Autodesk Inventor part; units mm, degrees
(part 4 of 4)
sketch "Sketch3" plane through (-107.46, -92.5006, 10.9251) normal (0, 0, 1) x (1, 0, 0)
  circle A0 centre (-216.125, 0) radius 1.35
  circle A1 centre (-216.125, 57) radius 1.35
  circle A2 centre (-216.125, -57) radius 1.35
  circle A3 centre (-216.125, 57) radius 1.35
  circle A4 centre (-216.125, 0) radius 1.35
  circle A5 centre (-216.125, -57) radius 1.35
  circle A6 centre (-175.75, 14.25) radius 1.35
  circle A7 centre (-175.75, -23.75) radius 1.35
  circle A8 centre (-133.753, -57) radius 1.35
  circle A9 centre (-114, 14.25) radius 1.35
  circle A10 centre (-73.625, 57) radius 1.35
  circle A11 centre (-66.5, -19) radius 1.35
  circle A12 centre (-47.5, -57) radius 1.35
  circle A13 centre (-45.125, 11.875) radius 1.35
  line L0 (-205.2313, 59.21) -> (-211.6644, 41.535)
  line L1 (-211.6644, 41.535) -> (-209.1644, 41.535)
  line L2 (-209.1644, 41.535) -> (-202.7313, 59.21)
  line L3 (-202.7313, 59.21) -> (-205.2313, 59.21)
  line L4 (-195.2313, 59.21) -> (-201.6644, 41.535)
  line L5 (-201.6644, 41.535) -> (-199.1644, 41.535)
  line L6 (-199.1644, 41.535) -> (-192.7313, 59.21)
  line L7 (-192.7313, 59.21) -> (-195.2313, 59.21)
  line L8 (-185.2313, 59.21) -> (-191.6644, 41.535)
  line L9 (-191.6644, 41.535) -> (-189.1644, 41.535)
  line L10 (-189.1644, 41.535) -> (-182.7313, 59.21)
  line L11 (-182.7313, 59.21) -> (-185.2313, 59.21)
  line L12 (-175.2313, 59.21) -> (-181.6644, 41.535)
  line L13 (-181.6644, 41.535) -> (-179.1644, 41.535)
  line L14 (-179.1644, 41.535) -> (-172.7313, 59.21)
  line L15 (-172.7313, 59.21) -> (-175.2313, 59.21)
  line L16 (-165.2313, 59.21) -> (-171.6644, 41.535)
  line L17 (-171.6644, 41.535) -> (-169.1644, 41.535)
  line L18 (-169.1644, 41.535) -> (-162.7313, 59.21)
  line L19 (-162.7313, 59.21) -> (-165.2313, 59.21)
  line L20 (-155.2313, 59.21) -> (-161.6644, 41.535)
  line L21 (-161.6644, 41.535) -> (-159.1644, 41.535)
  line L22 (-159.1644, 41.535) -> (-152.7313, 59.21)
  line L23 (-152.7313, 59.21) -> (-155.2313, 59.21)
  line L24 (-145.2313, 59.21) -> (-151.6644, 41.535)
  line L25 (-151.6644, 41.535) -> (-149.1644, 41.535)
  line L26 (-149.1644, 41.535) -> (-142.7313, 59.21)
  line L27 (-142.7313, 59.21) -> (-145.2313, 59.21)
  line L28 (-135.2313, 59.21) -> (-141.6644, 41.535)
  line L29 (-141.6644, 41.535) -> (-139.1644, 41.535)
  line L30 (-139.1644, 41.535) -> (-132.7313, 59.21)
  line L31 (-132.7313, 59.21) -> (-135.2313, 59.21)
  line L32 (-136.6647, 41.535) -> (-134.1647, 41.535)
  line L33 (-134.1647, 41.535) -> (-131.39, 49.1583)
  line L34 (-131.39, 49.1583) -> (-131.39, 56.027)
  line L35 (-131.39, 56.027) -> (-136.6647, 41.535)
  line L36 (-143.77, 35.75) -> (-141.27, 35.75)
  line L37 (-141.27, 35.75) -> (-139.8378, 39.685)
  line L38 (-139.8378, 39.685) -> (-142.3378, 39.685)
  line L39 (-142.3378, 39.685) -> (-143.77, 35.75)
  line L40 (-153.77, 35.75) -> (-151.27, 35.75)
  line L41 (-151.27, 35.75) -> (-149.8378, 39.685)
  line L42 (-149.8378, 39.685) -> (-152.3378, 39.685)
  line L43 (-152.3378, 39.685) -> (-153.77, 35.75)
  line L44 (-163.77, 35.75) -> (-161.27, 35.75)
  line L45 (-161.27, 35.75) -> (-159.8378, 39.685)
  line L46 (-159.8378, 39.685) -> (-162.3378, 39.685)
  line L47 (-162.3378, 39.685) -> (-163.77, 35.75)
  line L48 (-173.77, 35.75) -> (-171.27, 35.75)
  line L49 (-171.27, 35.75) -> (-169.8378, 39.685)
  line L50 (-169.8378, 39.685) -> (-172.3378, 39.685)
  line L51 (-172.3378, 39.685) -> (-173.77, 35.75)
  line L52 (-183.77, 35.75) -> (-181.27, 35.75)
  line L53 (-181.27, 35.75) -> (-179.8378, 39.685)
  line L54 (-179.8378, 39.685) -> (-182.3378, 39.685)
  line L55 (-182.3378, 39.685) -> (-183.77, 35.75)
  line L56 (-193.77, 35.75) -> (-191.27, 35.75)
  line L57 (-191.27, 35.75) -> (-189.8378, 39.685)
  line L58 (-189.8378, 39.685) -> (-192.3378, 39.685)
  line L59 (-192.3378, 39.685) -> (-193.77, 35.75)
  line L60 (-203.77, 35.75) -> (-201.27, 35.75)
  line L61 (-201.27, 35.75) -> (-199.8378, 39.685)
  line L62 (-199.8378, 39.685) -> (-202.3378, 39.685)
  line L63 (-202.3378, 39.685) -> (-203.77, 35.75)
  line L64 (-213.77, 35.75) -> (-211.27, 35.75)
  line L65 (-211.27, 35.75) -> (-209.8378, 39.685)
  line L66 (-209.8378, 39.685) -> (-212.3378, 39.685)
  line L67 (-212.3378, 39.685) -> (-213.77, 35.75)
  line L68 (-208.77, 35.75) -> (-206.27, 35.75)
  line L69 (-206.27, 35.75) -> (-204.8378, 39.685)
  line L70 (-204.8378, 39.685) -> (-207.3378, 39.685)
  line L71 (-207.3378, 39.685) -> (-208.77, 35.75)
  line L72 (-198.77, 35.75) -> (-196.27, 35.75)
  line L73 (-196.27, 35.75) -> (-194.8378, 39.685)
  line L74 (-194.8378, 39.685) -> (-197.3378, 39.685)
  line L75 (-197.3378, 39.685) -> (-198.77, 35.75)
  line L76 (-188.77, 35.75) -> (-186.27, 35.75)
  line L77 (-186.27, 35.75) -> (-184.8378, 39.685)
  line L78 (-184.8378, 39.685) -> (-187.3378, 39.685)
  line L79 (-187.3378, 39.685) -> (-188.77, 35.75)
  line L80 (-178.77, 35.75) -> (-176.27, 35.75)
  line L81 (-176.27, 35.75) -> (-174.8378, 39.685)
  line L82 (-174.8378, 39.685) -> (-177.3378, 39.685)
  line L83 (-177.3378, 39.685) -> (-178.77, 35.75)
  line L84 (-168.77, 35.75) -> (-166.27, 35.75)
  line L85 (-166.27, 35.75) -> (-164.8378, 39.685)
  line L86 (-164.8378, 39.685) -> (-167.3378, 39.685)
  line L87 (-167.3378, 39.685) -> (-168.77, 35.75)
  line L88 (-158.77, 35.75) -> (-156.27, 35.75)
  line L89 (-156.27, 35.75) -> (-154.8378, 39.685)
  line L90 (-154.8378, 39.685) -> (-157.3378, 39.685)
  line L91 (-157.3378, 39.685) -> (-158.77, 35.75)
  line L92 (-148.77, 35.75) -> (-146.27, 35.75)
  line L93 (-146.27, 35.75) -> (-144.8378, 39.685)
  line L94 (-144.8378, 39.685) -> (-147.3378, 39.685)
  line L95 (-147.3378, 39.685) -> (-148.77, 35.75)
  line L96 (-138.7702, 35.75) -> (-136.2702, 35.75)
  line L97 (-136.2702, 35.75) -> (-134.838, 39.685)
  line L98 (-134.838, 39.685) -> (-137.338, 39.685)
  line L99 (-137.338, 39.685) -> (-138.7702, 35.75)
  line L100 (-210.231, 59.21) -> (-213.77, 49.4867)
  line L101 (-213.77, 49.4867) -> (-213.77, 42.618)
  line L102 (-213.77, 42.618) -> (-207.731, 59.21)
  line L103 (-207.731, 59.21) -> (-210.231, 59.21)
  line L104 (-140.2313, 59.21) -> (-146.6644, 41.535)
  line L105 (-146.6644, 41.535) -> (-144.1644, 41.535)
  line L106 (-144.1644, 41.535) -> (-137.7313, 59.21)
  line L107 (-137.7313, 59.21) -> (-140.2313, 59.21)
  line L108 (-150.2313, 59.21) -> (-156.6644, 41.535)
  line L109 (-156.6644, 41.535) -> (-154.1644, 41.535)
  line L110 (-154.1644, 41.535) -> (-147.7313, 59.21)
  line L111 (-147.7313, 59.21) -> (-150.2313, 59.21)
  line L112 (-160.2313, 59.21) -> (-166.6644, 41.535)
  line L113 (-166.6644, 41.535) -> (-164.1644, 41.535)
  line L114 (-164.1644, 41.535) -> (-157.7313, 59.21)
  line L115 (-157.7313, 59.21) -> (-160.2313, 59.21)
  line L116 (-170.2313, 59.21) -> (-176.6644, 41.535)
  line L117 (-176.6644, 41.535) -> (-174.1644, 41.535)
  line L118 (-174.1644, 41.535) -> (-167.7313, 59.21)
  line L119 (-167.7313, 59.21) -> (-170.2313, 59.21)
  line L120 (-180.2313, 59.21) -> (-186.6644, 41.535)
  line L121 (-186.6644, 41.535) -> (-184.1644, 41.535)
  line L122 (-184.1644, 41.535) -> (-177.7313, 59.21)
  line L123 (-177.7313, 59.21) -> (-180.2313, 59.21)
  line L124 (-190.2313, 59.21) -> (-196.6644, 41.535)
  line L125 (-196.6644, 41.535) -> (-194.1644, 41.535)
  line L126 (-194.1644, 41.535) -> (-187.7313, 59.21)
  line L127 (-187.7313, 59.21) -> (-190.2313, 59.21)
  line L128 (-200.2313, 59.21) -> (-206.6644, 41.535)
  line L129 (-206.6644, 41.535) -> (-204.1644, 41.535)
  line L130 (-204.1644, 41.535) -> (-197.7313, 59.21)
  line L131 (-197.7313, 59.21) -> (-200.2313, 59.21)
  line L132 (-133.77, 35.75) -> (-78.7722, 35.75)
  line L133 (-78.7722, 35.75) -> (-77.34, 39.685)
  line L134 (-77.34, 39.685) -> (-132.3378, 39.685)
  line L135 (-132.3378, 39.685) -> (-133.77, 35.75)
  line L136 (-216.125, 61.75) -> (216.125, 61.75)
  arc A14 (220.875, 57) -> (216.125, 61.75) centre (216.125, 57) ccw
  line L137 (220.875, 57) -> (220.875, -57)
  arc A15 (216.125, -61.75) -> (220.875, -57) centre (216.125, -57) ccw
  line L138 (216.125, -61.75) -> (-216.125, -61.75)
  arc A16 (-220.875, -57) -> (-216.125, -61.75) centre (-216.125, -57) ccw
  line L139 (-220.875, -57) -> (-220.875, 57)
  arc A17 (-216.125, 61.75) -> (-220.875, 57) centre (-216.125, 57) ccw
  line L140 (-129.54, 41.535) -> (-77.34, 41.535)
  line L141 (-77.34, 41.535) -> (-77.34, 59.315)
  line L142 (-77.34, 59.315) -> (-129.54, 59.315)
  line L143 (-129.54, 59.315) -> (-129.54, 41.535)
  line L144 (-54.75, 45.25) -> (-54.75, 59.25)
  line L145 (-54.75, 59.25) -> (-68.75, 59.25)
  line L146 (-68.75, 59.25) -> (-68.75, 45.25)
  line L147 (-68.75, 45.25) -> (-54.75, 45.25)
  line L148 (-16.75, 45.25) -> (-16.75, 59.25)
  line L149 (-16.75, 59.25) -> (-30.75, 59.25)
  line L150 (-30.75, 59.25) -> (-30.75, 45.25)
  line L151 (-30.75, 45.25) -> (-16.75, 45.25)
  line L152 (2.25, 45.25) -> (2.25, 59.25)
  line L153 (2.25, 59.25) -> (-11.75, 59.25)
  line L154 (-11.75, 59.25) -> (-11.75, 45.25)
  line L155 (-11.75, 45.25) -> (2.25, 45.25)
  line L156 (21.25, 45.25) -> (21.25, 59.25)
  line L157 (21.25, 59.25) -> (7.25, 59.25)
  line L158 (7.25, 59.25) -> (7.25, 45.25)
  line L159 (7.25, 45.25) -> (21.25, 45.25)
  line L160 (40.25, 45.25) -> (40.25, 59.25)
  line L161 (40.25, 59.25) -> (26.25, 59.25)
  line L162 (26.25, 59.25) -> (26.25, 45.25)
  line L163 (26.25, 45.25) -> (40.25, 45.25)
  line L164 (68.75, 45.25) -> (68.75, 59.25)
  line L165 (68.75, 59.25) -> (54.75, 59.25)
  line L166 (54.75, 59.25) -> (54.75, 45.25)
  line L167 (54.75, 45.25) -> (68.75, 45.25)
  line L168 (87.75, 45.25) -> (87.75, 59.25)
  line L169 (87.75, 59.25) -> (73.75, 59.25)
  line L170 (73.75, 59.25) -> (73.75, 45.25)
  line L171 (73.75, 45.25) -> (87.75, 45.25)
  line L172 (106.75, 45.25) -> (106.75, 59.25)
  line L173 (106.75, 59.25) -> (92.75, 59.25)
  line L174 (92.75, 59.25) -> (92.75, 45.25)
  line L175 (92.75, 45.25) -> (106.75, 45.25)
  line L176 (125.75, 45.25) -> (125.75, 59.25)
  line L177 (125.75, 59.25) -> (111.75, 59.25)
  line L178 (111.75, 59.25) -> (111.75, 45.25)
  line L179 (111.75, 45.25) -> (125.75, 45.25)
  line L180 (154.25, 45.25) -> (154.25, 59.25)
  line L181 (154.25, 59.25) -> (140.25, 59.25)
  line L182 (140.25, 59.25) -> (140.25, 45.25)
  line L183 (140.25, 45.25) -> (154.25, 45.25)
  line L184 (173.25, 45.25) -> (173.25, 59.25)
  line L185 (173.25, 59.25) -> (159.25, 59.25)
  line L186 (159.25, 59.25) -> (159.25, 45.25)
  line L187 (159.25, 45.25) -> (173.25, 45.25)
  line L188 (192.25, 45.25) -> (192.25, 59.25)
  line L189 (192.25, 59.25) -> (178.25, 59.25)
  line L190 (178.25, 59.25) -> (178.25, 45.25)
  line L191 (178.25, 45.25) -> (192.25, 45.25)
  line L192 (211.25, 45.25) -> (211.25, 59.25)
  line L193 (211.25, 59.25) -> (197.25, 59.25)
  line L194 (197.25, 59.25) -> (197.25, 45.25)
  line L195 (197.25, 45.25) -> (211.25, 45.25)
  line L196 (-197.25, 16.75) -> (-197.25, 30.75)
  line L197 (-197.25, 30.75) -> (-211.25, 30.75)
  line L198 (-211.25, 30.75) -> (-211.25, 16.75)
  line L199 (-211.25, 16.75) -> (-197.25, 16.75)
  line L200 (-178.25, 30.75) -> (-192.25, 30.75)
  line L201 (-192.25, 30.75) -> (-192.25, 16.75)
  line L202 (-192.25, 16.75) -> (-178.25, 16.75)
  line L203 (-178.25, 16.75) -> (-178.25, 30.75)
  line L204 (-159.25, 30.75) -> (-173.25, 30.75)
  line L205 (-173.25, 30.75) -> (-173.25, 16.75)
  line L206 (-173.25, 16.75) -> (-159.25, 16.75)
  line L207 (-159.25, 16.75) -> (-159.25, 30.75)
  line L208 (-197.25, 11.75) -> (-211.25, 11.75)
  line L209 (-211.25, 11.75) -> (-211.25, -2.25)
  line L210 (-211.25, -2.25) -> (-197.25, -2.25)
  line L211 (-197.25, -2.25) -> (-197.25, 11.75)
  line L212 (-178.25, 11.75) -> (-192.25, 11.75)
  line L213 (-192.25, 11.75) -> (-192.25, -2.25)
  line L214 (-192.25, -2.25) -> (-178.25, -2.25)
  line L215 (-178.25, -2.25) -> (-178.25, 11.75)
  line L216 (-159.25, 11.75) -> (-173.25, 11.75)
  line L217 (-173.25, 11.75) -> (-173.25, -2.25)
  line L218 (-173.25, -2.25) -> (-159.25, -2.25)
  line L219 (-159.25, -2.25) -> (-159.25, 11.75)
  line L220 (-197.25, -7.25) -> (-211.25, -7.25)
  line L221 (-211.25, -7.25) -> (-211.25, -21.25)
  line L222 (-211.25, -21.25) -> (-197.25, -21.25)
  line L223 (-197.25, -21.25) -> (-197.25, -7.25)
  line L224 (-178.25, -7.25) -> (-192.25, -7.25)
  line L225 (-192.25, -7.25) -> (-192.25, -21.25)
  line L226 (-192.25, -21.25) -> (-178.25, -21.25)
  line L227 (-178.25, -21.25) -> (-178.25, -7.25)
  line L228 (-159.25, -7.25) -> (-173.25, -7.25)
  line L229 (-173.25, -7.25) -> (-173.25, -21.25)
  line L230 (-173.25, -21.25) -> (-159.25, -21.25)
  line L231 (-159.25, -21.25) -> (-159.25, -7.25)
  line L232 (-197.25, -26.25) -> (-211.25, -26.25)
  line L233 (-211.25, -26.25) -> (-211.25, -40.25)
  line L234 (-211.25, -40.25) -> (-197.25, -40.25)
  line L235 (-197.25, -40.25) -> (-197.25, -26.25)
  line L236 (-178.25, -26.25) -> (-192.25, -26.25)
  line L237 (-192.25, -26.25) -> (-192.25, -40.25)
  line L238 (-192.25, -40.25) -> (-178.25, -40.25)
  line L239 (-178.25, -40.25) -> (-178.25, -26.25)
  line L240 (-159.25, -26.25) -> (-173.25, -26.25)
  line L241 (-173.25, -26.25) -> (-173.25, -40.25)
  line L242 (-173.25, -40.25) -> (-159.25, -40.25)
  line L243 (-159.25, -40.25) -> (-159.25, -26.25)
  line L244 (-197.25, -45.25) -> (-211.25, -45.25)
  line L245 (-211.25, -45.25) -> (-211.25, -59.25)
  line L246 (-211.25, -59.25) -> (-197.25, -59.25)
  line L247 (-197.25, -59.25) -> (-197.25, -45.25)
  line L248 (-178.25, -45.25) -> (-192.25, -45.25)
  line L249 (-192.25, -45.25) -> (-192.25, -59.25)
  line L250 (-192.25, -59.25) -> (-178.25, -59.25)
  line L251 (-178.25, -59.25) -> (-178.25, -45.25)
  line L252 (-159.25, -45.25) -> (-173.25, -45.25)
  line L253 (-173.25, -45.25) -> (-173.25, -59.25)
  line L254 (-173.25, -59.25) -> (-159.25, -59.25)
  line L255 (-159.25, -59.25) -> (-159.25, -45.25)
  line L256 (-140.25, 16.75) -> (-140.25, 30.75)
  line L257 (-140.25, 30.75) -> (-154.25, 30.75)
  line L258 (-154.25, 30.75) -> (-154.25, 16.75)
  line L259 (-154.25, 16.75) -> (-140.25, 16.75)
  line L260 (-140.25, -11.75) -> (-140.25, 2.25)
  line L261 (-140.25, 2.25) -> (-154.25, 2.25)
  line L262 (-154.25, 2.25) -> (-154.25, -11.75)
  line L263 (-154.25, -11.75) -> (-140.25, -11.75)
  line L264 (-140.25, -49.75) -> (-140.25, -35.75)
  line L265 (-140.25, -35.75) -> (-154.25, -35.75)
  line L266 (-154.25, -35.75) -> (-154.25, -49.75)
  line L267 (-154.25, -49.75) -> (-140.25, -49.75)
  line L268 (-116.5, -59.25) -> (-116.5, -45.25)
  line L269 (-116.5, -45.25) -> (-130.5, -45.25)
  line L270 (-130.5, -45.25) -> (-130.5, -59.25)
  line L271 (-130.5, -59.25) -> (-116.5, -59.25)
  line L272 (-97.5, -59.25) -> (-97.5, -45.25)
  line L273 (-97.5, -45.25) -> (-111.5, -45.25)
  line L274 (-111.5, -45.25) -> (-111.5, -59.25)
  line L275 (-111.5, -59.25) -> (-97.5, -59.25)
  line L276 (-78.5, -59.25) -> (-78.5, -45.25)
  line L277 (-78.5, -45.25) -> (-92.5, -45.25)
  line L278 (-92.5, -45.25) -> (-92.5, -59.25)
  line L279 (-92.5, -59.25) -> (-78.5, -59.25)
  line L280 (-97.5, -40.25) -> (-97.5, -26.25)
  line L281 (-97.5, -26.25) -> (-111.5, -26.25)
  line L282 (-111.5, -26.25) -> (-111.5, -40.25)
  line L283 (-111.5, -40.25) -> (-97.5, -40.25)
  line L284 (-116.5, 16.75) -> (-116.5, 30.75)
  line L285 (-116.5, 30.75) -> (-130.5, 30.75)
  line L286 (-130.5, 30.75) -> (-130.5, 16.75)
  line L287 (-130.5, 16.75) -> (-116.5, 16.75)
  line L288 (-111.5, 30.75) -> (-111.5, 16.75)
  line L289 (-111.5, 16.75) -> (-97.5, 16.75)
  line L290 (-97.5, 16.75) -> (-97.5, 30.75)
  line L291 (-97.5, 30.75) -> (-111.5, 30.75)
  line L292 (-92.5, 30.75) -> (-92.5, 16.75)
  line L293 (-92.5, 16.75) -> (-78.5, 16.75)
  line L294 (-78.5, 16.75) -> (-78.5, 30.75)
  line L295 (-78.5, 30.75) -> (-92.5, 30.75)
  line L296 (-130.5, 11.75) -> (-130.5, -2.25)
  line L297 (-130.5, -2.25) -> (-116.5, -2.25)
  line L298 (-116.5, -2.25) -> (-116.5, 11.75)
  line L299 (-116.5, 11.75) -> (-130.5, 11.75)
  line L300 (-111.5, 11.75) -> (-111.5, -2.25)
  line L301 (-111.5, -2.25) -> (-97.5, -2.25)
  line L302 (-97.5, -2.25) -> (-97.5, 11.75)
  line L303 (-97.5, 11.75) -> (-111.5, 11.75)
  line L304 (-92.5, 11.75) -> (-92.5, -2.25)
  line L305 (-92.5, -2.25) -> (-78.5, -2.25)
  line L306 (-78.5, -2.25) -> (-78.5, 11.75)
  line L307 (-78.5, 11.75) -> (-92.5, 11.75)
  line L308 (-54.75, 16.75) -> (-54.75, 30.75)
  line L309 (-54.75, 30.75) -> (-68.75, 30.75)
  line L310 (-68.75, 30.75) -> (-68.75, 16.75)
  line L311 (-68.75, 16.75) -> (-54.75, 16.75)
  line L312 (-35.75, 16.75) -> (-35.75, 30.75)
  line L313 (-35.75, 30.75) -> (-49.75, 30.75)
  line L314 (-49.75, 30.75) -> (-49.75, 16.75)
  line L315 (-49.75, 16.75) -> (-35.75, 16.75)
  line L316 (-16.75, 16.75) -> (-16.75, 30.75)
  line L317 (-16.75, 30.75) -> (-30.75, 30.75)
  line L318 (-30.75, 30.75) -> (-30.75, 16.75)
  line L319 (-30.75, 16.75) -> (-16.75, 16.75)
  line L320 (2.25, 16.75) -> (2.25, 30.75)
  line L321 (2.25, 30.75) -> (-11.75, 30.75)
  line L322 (-11.75, 30.75) -> (-11.75, 16.75)
  line L323 (-11.75, 16.75) -> (2.25, 16.75)
  line L324 (21.25, 16.75) -> (21.25, 30.75)
  line L325 (21.25, 30.75) -> (7.25, 30.75)
  line L326 (7.25, 30.75) -> (7.25, 16.75)
  line L327 (7.25, 16.75) -> (21.25, 16.75)
  line L328 (40.25, 16.75) -> (40.25, 30.75)
  line L329 (40.25, 30.75) -> (26.25, 30.75)
  line L330 (26.25, 30.75) -> (26.25, 16.75)
  line L331 (26.25, 16.75) -> (40.25, 16.75)
  line L332 (59.25, 16.75) -> (59.25, 30.75)
  line L333 (59.25, 30.75) -> (45.25, 30.75)
  line L334 (45.25, 30.75) -> (45.25, 16.75)
  line L335 (45.25, 16.75) -> (59.25, 16.75)
  line L336 (78.25, 16.75) -> (78.25, 30.75)
  line L337 (78.25, 30.75) -> (64.25, 30.75)
  line L338 (64.25, 30.75) -> (64.25, 16.75)
  line L339 (64.25, 16.75) -> (78.25, 16.75)
  line L340 (97.25, 16.75) -> (97.25, 30.75)
  line L341 (97.25, 30.75) -> (83.25, 30.75)
  line L342 (83.25, 30.75) -> (83.25, 16.75)
  line L343 (83.25, 16.75) -> (97.25, 16.75)
  line L344 (116.25, 16.75) -> (116.25, 30.75)
  line L345 (116.25, 30.75) -> (102.25, 30.75)
  line L346 (102.25, 30.75) -> (102.25, 16.75)
  line L347 (102.25, 16.75) -> (116.25, 16.75)
  line L348 (135.25, 16.75) -> (135.25, 30.75)
  line L349 (135.25, 30.75) -> (121.25, 30.75)
  line L350 (121.25, 30.75) -> (121.25, 16.75)
  line L351 (121.25, 16.75) -> (135.25, 16.75)
  line L352 (154.25, 16.75) -> (154.25, 30.75)
  line L353 (154.25, 30.75) -> (140.25, 30.75)
  line L354 (140.25, 30.75) -> (140.25, 16.75)
  line L355 (140.25, 16.75) -> (154.25, 16.75)
  line L356 (173.25, 16.75) -> (173.25, 30.75)
  line L357 (173.25, 30.75) -> (159.25, 30.75)
  line L358 (159.25, 30.75) -> (159.25, 16.75)
  line L359 (159.25, 16.75) -> (173.25, 16.75)
  line L360 (-50, -2.25) -> (-50, 11.75)
  line L361 (-50, 11.75) -> (-64, 11.75)
  line L362 (-64, 11.75) -> (-64, -2.25)
  line L363 (-64, -2.25) -> (-50, -2.25)
  line L364 (-47.625, -21.25) -> (-47.625, -7.25)
  line L365 (-47.625, -7.25) -> (-61.625, -7.25)
  line L366 (-61.625, -7.25) -> (-61.625, -21.25)
  line L367 (-61.625, -21.25) -> (-47.625, -21.25)
  line L368 (-42.875, -40.25) -> (-42.875, -26.25)
  line L369 (-42.875, -26.25) -> (-56.875, -26.25)
  line L370 (-56.875, -26.25) -> (-56.875, -40.25)
  line L371 (-56.875, -40.25) -> (-42.875, -40.25)
  line L372 (-52.375, -59.25) -> (-52.375, -45.25)
  line L373 (-52.375, -45.25) -> (-66.375, -45.25)
  line L374 (-66.375, -45.25) -> (-66.375, -59.25)
  line L375 (-66.375, -59.25) -> (-52.375, -59.25)
  line L376 (-28.625, -59.25) -> (-28.625, -45.25)
  line L377 (-28.625, -45.25) -> (-42.625, -45.25)
  line L378 (-42.625, -45.25) -> (-42.625, -59.25)
  line L379 (-42.625, -59.25) -> (-28.625, -59.25)
  line L380 (-4.875, -59.25) -> (-4.875, -45.25)
  line L381 (-4.875, -45.25) -> (-18.875, -45.25)
  line L382 (-18.875, -45.25) -> (-18.875, -59.25)
  line L383 (-18.875, -59.25) -> (-4.875, -59.25)
  line L384 (78.25, -59.25) -> (78.25, -45.25)
  line L385 (78.25, -45.25) -> (64.25, -45.25)
  line L386 (64.25, -45.25) -> (64.25, -59.25)
  line L387 (64.25, -59.25) -> (78.25, -59.25)
  line L388 (161.375, -59.25) -> (161.375, -45.25)
  line L389 (161.375, -45.25) -> (147.375, -45.25)
  line L390 (147.375, -45.25) -> (147.375, -59.25)
  line L391 (147.375, -59.25) -> (161.375, -59.25)
  line L392 (185.125, -59.25) -> (185.125, -45.25)
  line L393 (185.125, -45.25) -> (171.125, -45.25)
  line L394 (171.125, -45.25) -> (171.125, -59.25)
  line L395 (171.125, -59.25) -> (185.125, -59.25)
  line L396 (208.875, -59.25) -> (208.875, -45.25)
  line L397 (208.875, -45.25) -> (194.875, -45.25)
  line L398 (194.875, -45.25) -> (194.875, -59.25)
  line L399 (194.875, -59.25) -> (208.875, -59.25)
  line L400 (194.625, -40.25) -> (194.625, -26.25)
  line L401 (194.625, -26.25) -> (180.625, -26.25)
  line L402 (180.625, -26.25) -> (180.625, -40.25)
  line L403 (180.625, -40.25) -> (194.625, -40.25)
  line L404 (199.375, -21.25) -> (199.375, -7.25)
  line L405 (199.375, -7.25) -> (185.375, -7.25)
  line L406 (185.375, -7.25) -> (185.375, -21.25)
  line L407 (185.375, -21.25) -> (199.375, -21.25)
  line L408 (206.5, -2.25) -> (206.5, 11.75)
  line L409 (206.5, 11.75) -> (192.5, 11.75)
  line L410 (192.5, 11.75) -> (192.5, -2.25)
  line L411 (192.5, -2.25) -> (206.5, -2.25)
  line L412 (201.75, 16.75) -> (201.75, 30.75)
  line L413 (201.75, 30.75) -> (187.75, 30.75)
  line L414 (187.75, 30.75) -> (187.75, 16.75)
  line L415 (187.75, 16.75) -> (201.75, 16.75)
  line L416 (-26.25, -2.25) -> (-26.25, 11.75)
  line L417 (-26.25, 11.75) -> (-40.25, 11.75)
  line L418 (-40.25, 11.75) -> (-40.25, -2.25)
  line L419 (-40.25, -2.25) -> (-26.25, -2.25)
  line L420 (-21.5, -21.25) -> (-21.5, -7.25)
  line L421 (-21.5, -7.25) -> (-35.5, -7.25)
  line L422 (-35.5, -7.25) -> (-35.5, -21.25)
  line L423 (-35.5, -21.25) -> (-21.5, -21.25)
  line L424 (-12, -40.25) -> (-12, -26.25)
  line L425 (-12, -26.25) -> (-26, -26.25)
  line L426 (-26, -26.25) -> (-26, -40.25)
  line L427 (-26, -40.25) -> (-12, -40.25)
  line L428 (-7.25, -2.25) -> (-7.25, 11.75)
  line L429 (-7.25, 11.75) -> (-21.25, 11.75)
  line L430 (-21.25, 11.75) -> (-21.25, -2.25)
  line L431 (-21.25, -2.25) -> (-7.25, -2.25)
  line L432 (11.75, -2.25) -> (11.75, 11.75)
  line L433 (11.75, 11.75) -> (-2.25, 11.75)
  line L434 (-2.25, 11.75) -> (-2.25, -2.25)
  line L435 (-2.25, -2.25) -> (11.75, -2.25)
  line L436 (30.75, -2.25) -> (30.75, 11.75)
  line L437 (30.75, 11.75) -> (16.75, 11.75)
  line L438 (16.75, 11.75) -> (16.75, -2.25)
  line L439 (16.75, -2.25) -> (30.75, -2.25)
  line L440 (49.75, -2.25) -> (49.75, 11.75)
  line L441 (49.75, 11.75) -> (35.75, 11.75)
  line L442 (35.75, 11.75) -> (35.75, -2.25)
  line L443 (35.75, -2.25) -> (49.75, -2.25)
  line L444 (68.75, -2.25) -> (68.75, 11.75)
  line L445 (68.75, 11.75) -> (54.75, 11.75)
  line L446 (54.75, 11.75) -> (54.75, -2.25)
  line L447 (54.75, -2.25) -> (68.75, -2.25)
  line L448 (87.75, -2.25) -> (87.75, 11.75)
  line L449 (87.75, 11.75) -> (73.75, 11.75)
  line L450 (73.75, 11.75) -> (73.75, -2.25)
  line L451 (73.75, -2.25) -> (87.75, -2.25)
  line L452 (106.75, -2.25) -> (106.75, 11.75)
  line L453 (106.75, 11.75) -> (92.75, 11.75)
  line L454 (92.75, 11.75) -> (92.75, -2.25)
  line L455 (92.75, -2.25) -> (106.75, -2.25)
  line L456 (125.75, -2.25) -> (125.75, 11.75)
  line L457 (125.75, 11.75) -> (111.75, 11.75)
  line L458 (111.75, 11.75) -> (111.75, -2.25)
  line L459 (111.75, -2.25) -> (125.75, -2.25)
  line L460 (144.75, -2.25) -> (144.75, 11.75)
  line L461 (144.75, 11.75) -> (130.75, 11.75)
  line L462 (130.75, 11.75) -> (130.75, -2.25)
  line L463 (130.75, -2.25) -> (144.75, -2.25)
  line L464 (163.75, -2.25) -> (163.75, 11.75)
  line L465 (163.75, 11.75) -> (149.75, 11.75)
  line L466 (149.75, 11.75) -> (149.75, -2.25)
  line L467 (149.75, -2.25) -> (163.75, -2.25)
  line L468 (182.75, -2.25) -> (182.75, 11.75)
  line L469 (182.75, 11.75) -> (168.75, 11.75)
  line L470 (168.75, 11.75) -> (168.75, -2.25)
  line L471 (168.75, -2.25) -> (182.75, -2.25)
  line L472 (-2.5, -7.25) -> (-16.5, -7.25)
  line L473 (-16.5, -7.25) -> (-16.5, -21.25)
  line L474 (-16.5, -21.25) -> (-2.5, -21.25)
  line L475 (-2.5, -21.25) -> (-2.5, -7.25)
  line L476 (16.5, -7.25) -> (2.5, -7.25)
  line L477 (2.5, -7.25) -> (2.5, -21.25)
  line L478 (2.5, -21.25) -> (16.5, -21.25)
  line L479 (16.5, -21.25) -> (16.5, -7.25)
  line L480 (35.5, -7.25) -> (21.5, -7.25)
  line L481 (21.5, -7.25) -> (21.5, -21.25)
  line L482 (21.5, -21.25) -> (35.5, -21.25)
  line L483 (35.5, -21.25) -> (35.5, -7.25)
  line L484 (54.5, -7.25) -> (40.5, -7.25)
  line L485 (40.5, -7.25) -> (40.5, -21.25)
  line L486 (40.5, -21.25) -> (54.5, -21.25)
  line L487 (54.5, -21.25) -> (54.5, -7.25)
  line L488 (73.5, -7.25) -> (59.5, -7.25)
  line L489 (59.5, -7.25) -> (59.5, -21.25)
  line L490 (59.5, -21.25) -> (73.5, -21.25)
  line L491 (73.5, -21.25) -> (73.5, -7.25)
  line L492 (92.5, -7.25) -> (78.5, -7.25)
  line L493 (78.5, -7.25) -> (78.5, -21.25)
  line L494 (78.5, -21.25) -> (92.5, -21.25)
  line L495 (92.5, -21.25) -> (92.5, -7.25)
  line L496 (111.5, -7.25) -> (97.5, -7.25)
  line L497 (97.5, -7.25) -> (97.5, -21.25)
  line L498 (97.5, -21.25) -> (111.5, -21.25)
  line L499 (111.5, -21.25) -> (111.5, -7.25)
  line L500 (130.5, -7.25) -> (116.5, -7.25)
  line L501 (116.5, -7.25) -> (116.5, -21.25)
  line L502 (116.5, -21.25) -> (130.5, -21.25)
  line L503 (130.5, -21.25) -> (130.5, -7.25)
  line L504 (149.5, -7.25) -> (135.5, -7.25)
  line L505 (135.5, -7.25) -> (135.5, -21.25)
  line L506 (135.5, -21.25) -> (149.5, -21.25)
  line L507 (149.5, -21.25) -> (149.5, -7.25)
  line L508 (168.5, -7.25) -> (154.5, -7.25)
  line L509 (154.5, -7.25) -> (154.5, -21.25)
  line L510 (154.5, -21.25) -> (168.5, -21.25)
  line L511 (168.5, -21.25) -> (168.5, -7.25)
  line L512 (7, -40.25) -> (7, -26.25)
  line L513 (7, -26.25) -> (-7, -26.25)
  line L514 (-7, -26.25) -> (-7, -40.25)
  line L515 (-7, -40.25) -> (7, -40.25)
  line L516 (26, -40.25) -> (26, -26.25)
  line L517 (26, -26.25) -> (12, -26.25)
  line L518 (12, -26.25) -> (12, -40.25)
  line L519 (12, -40.25) -> (26, -40.25)
  line L520 (45, -40.25) -> (45, -26.25)
  line L521 (45, -26.25) -> (31, -26.25)
  line L522 (31, -26.25) -> (31, -40.25)
  line L523 (31, -40.25) -> (45, -40.25)
  line L524 (64, -40.25) -> (64, -26.25)
  line L525 (64, -26.25) -> (50, -26.25)
  line L526 (50, -26.25) -> (50, -40.25)
  line L527 (50, -40.25) -> (64, -40.25)
  line L528 (83, -40.25) -> (83, -26.25)
  line L529 (83, -26.25) -> (69, -26.25)
  line L530 (69, -26.25) -> (69, -40.25)
  line L531 (69, -40.25) -> (83, -40.25)
  line L532 (102, -40.25) -> (102, -26.25)
  line L533 (102, -26.25) -> (88, -26.25)
  line L534 (88, -26.25) -> (88, -40.25)
  line L535 (88, -40.25) -> (102, -40.25)
  line L536 (121, -40.25) -> (121, -26.25)
  line L537 (121, -26.25) -> (107, -26.25)
  line L538 (107, -26.25) -> (107, -40.25)
  line L539 (107, -40.25) -> (121, -40.25)
  line L540 (140, -40.25) -> (140, -26.25)
  line L541 (140, -26.25) -> (126, -26.25)
  line L542 (126, -26.25) -> (126, -40.25)
  line L543 (126, -40.25) -> (140, -40.25)
  line L544 (159, -40.25) -> (159, -26.25)
  line L545 (159, -26.25) -> (145, -26.25)
  line L546 (145, -26.25) -> (145, -40.25)
  line L547 (145, -40.25) -> (159, -40.25)
  circle A18 centre (-9.5, -24.356) radius 1.35
  circle A19 centre (23.75, -57) radius 1.35
  circle A20 centre (33.25, 13.49) radius 1.35
  circle A21 centre (47.5, 57) radius 1.35
  circle A22 centre (76, -23.086) radius 1.35
  circle A23 centre (109.25, 13.49) radius 1.35
  circle A24 centre (118.75, -57) radius 1.35
  circle A25 centre (133, 57) radius 1.35
  circle A26 centre (166.25, -40.375) radius 1.35
  circle A27 centre (187.625, 11.875) radius 1.35
  circle A28 centre (187.625, 11.875) radius 1.35
  circle A29 centre (216.125, 57) radius 1.35
  circle A30 centre (216.125, 0) radius 1.35
  circle A31 centre (216.125, -57) radius 1.35
  point P0 (107.46, 92.5006)
hole "Hole1" at (-323.585, -35.5006, 10.9251) at (-323.585, -92.5006, 10.9251) at (-323.585, -149.5006, 10.9251) at (-241.213, -149.5006, 10.9251) at (-173.96, -111.5006, 10.9251) at (-154.96, -149.5006, 10.9251) at (-83.71, -149.5006, 10.9251) at (-152.585, -80.6256, 10.9251) at (-181.085, -35.5006, 10.9251) at (-74.21, -79.0106, 10.9251) at (-59.96, -35.5006, 10.9251) at (-31.46, -115.5866, 10.9251) at (11.29, -149.5006, 10.9251) at (58.79, -132.8756, 10.9251) at (108.665, -92.5006, 10.9251) at (80.165, -80.6256, 10.9251) at (25.54, -35.5006, 10.9251) at (108.665, -35.5006, 10.9251) at (108.665, -149.5006, 10.9251) at (-221.46, -78.2506, 10.9251) at (-283.21, -78.2506, 10.9251) at (-283.21, -116.2506, 10.9251) at (1.79, -79.0106, 10.9251) at (-116.96, -116.8566, 10.9251) direction (0, 0, -1) diameter 2.5 depth 8 countersink diameter 4.7 countersink angle 90
body "Solid1"
